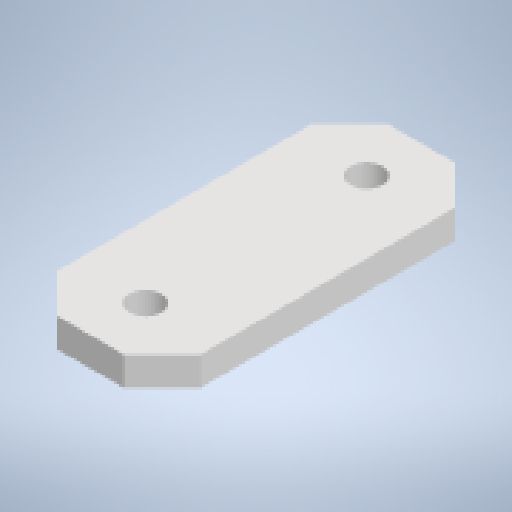
# Autodesk Inventor part: A1_joiners
Saved by Autodesk Inventor 2025.2 (Build 292293000, 293)
## iProperties
Created: 2025-03-24
Part Number: A1_joiners
Material: Generic
Document SubType Name: Sheet Metal
Designer: Caspe
Density: 1 g/cm^3
Sheet Metal Rule: Default_mm
Appearance: Default
Author: Caspe
Autodesk Inventor part; units mm, degrees
ref_plane "YZ Plane" through (0, 0, 0) normal (1, 0, 0) x (0, 1, 0)
ref_plane "XZ Plane" through (0, 0, 0) normal (0, 1, 0) x (-1, 0, 0)
ref_plane "XY Plane" through (0, 0, 0) normal (0, 0, 1) x (1, 0, 0)
sketch "Sketch1" plane through (0, 0, 0) normal (0, 1, 0) x (-1, 0, 0)
  line L0 (0, 0) -> (15, 0)
  line L1 (15, 0) -> (15, -34.5)
  line L2 (15, -34.5) -> (0, -34.5)
  line L3 (0, -34.5) -> (0, 0)
  line L4 (0, -17.25) -> (15, -17.25)
  circle A0 centre (7.5, -5.75) radius 1.675
  circle A1 centre (7.5, -28.75) radius 1.675
  circle A2 centre (-42.5, -5.75) radius 1.675
  line L5 (15, 0) -> (-50, 0)
  line L6 (-50, 0) -> (-50, -34.5)
  line L7 (-50, -34.5) -> (15, -34.5)
  line L8 (15, -34.5) -> (15, 0)
  circle A3 centre (-42.5, -28.75) radius 1.675
  point P0 (0, -34.5)
  dimension "d0" = 34.5
  dimension "d1" = 15
  dimension "d2" = 3.35
  dimension "d3" = 7.5
  dimension "d4" = 11.5
  dimension "d9" = 3.35
  dimension "d10" = 50
  dimension "d11" = 7.5
  dimension "d12" = 5.75
  measures "d0" distance of L0.end L1.end
  measures "d1" distance between parallel lines of L3 L1
  measures "d2" diameter of A0
  measures "d3" distance from line of L3 A0.centre
  measures "d4" distance from line of L4 A0.centre
  measures "d9" diameter of A2
  measures "d10" distance of A2.centre A0.centre
  measures "d11" distance from line of L6 A2.centre
  measures "d12" distance from line of L5 A2.centre
extrude "Plate1" add sketch "Sketch1" along normal blind 3
chamfer "Corner Chamfer1" distance 4 angle 45 4 edges at (-15, 1.5, 0) (-15, 1.5, -34.5) (50, 1.5, 0) (50, 1.5, -34.5)
equation "\"d0\" = 0.75 * A_width"
equation "\"d2\" = rivet_diameter"
equation "\"d3\" = 0.5 * d1"
equation "\"d4\" = 0.25 * A_width"
equation "\"d9\" = rivet_diameter"
equation "\"d5\" = Thickness"
equation "\"Thickness\" = plate_thickness"
equation "\"BendRadius\" = Thickness"
equation "\"BendReliefWidth\" = Thickness"
equation "\"BendReliefDepth\" = 0.5 * Thickness"
equation "\"CornerReliefSize\" = 4 * Thickness"
equation "\"MinimumRemnant\" = 2 * Thickness"
equation "\"TransitionRadius\" = BendRadius"
equation "\"JacobiRadiusSize\" = BendRadius"
equation "\"GapSize\" = Thickness"
equation "\"A_width\" = 46"
equation "\"A_joint_diameter\" = 16"
equation "\"A_joint_tolerance\" = 3"
equation "\"l___________\" = 0"
equation "\"l__________\" = 0"
equation "\"l_________\" = 0"
equation "\"rivet_diameter\" = 3.35"
equation "\"plate_thickness\" = 3"
equation "\"l________\" = 0"
equation "\"A_B_spacing\" = 2"
equation "\"L_Piston_Bottom\" = 21"
equation "\"L_Piston_Top\" = 25"
equation "\"thin_plate\" = 1.5"
body "Solid1"
